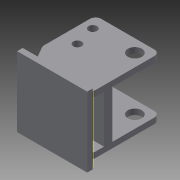
# Autodesk Inventor part: kepala 1 revisi
Saved by Autodesk Inventor 2014 SP2 (Build 180246200, 246)
## iProperties
Created: 2019-06-26
Part Number: kepala 1 revisi
Material: Generic
Document SubType Name: Modeling
Designer: USER PC
Density: 1 g/cm^3
Appearance: Default
Author: USER PC
Autodesk Inventor part; units mm, degrees
ref_plane "YZ Plane" through (0, 0, 0) normal (1, 0, 0) x (0, 1, 0)
ref_plane "XY Plane" through (0, 0, 0) normal (0, 0, 1) x (1, 0, 0)
sketch "Sketch1" plane through (0, 0, 0) normal (0, 0, 1) x (1, 0, 0)
  circle A0 centre (0, 0) radius 15
  circle A1 centre (150, 0) radius 25
  line L0 (-35, 45) -> (-35, -144.3782)
  circle A2 centre (20.0962, -75) radius 15
  line L1 (195, 45) -> (-35, 45)
  line L2 (195, -205) -> (0, -205)
  line L3 (195, -205) -> (195, 45)
  line L4 (0, -205) -> (-35, -144.3782)
  line L5 (0, -205) -> (70, -205) construction
  dimension "d0" = 230
  dimension "d1" = 120
  constraints: 12 end point, 3 centre point, 1 coincident, 1 equal length, 1 horizontal, 1 parallel, 1 perpendicular
  measures "d0" distance of L1.start L0.start
  measures "d1" angle of L5 L4
extrude "Extrusion1" add sketch "Sketch1" along normal blind 210
fillet "Fillet1" radius 20 1 edges at (195, 45, 105)
fillet "Fillet2" radius 20 1 edges at (195, -205, 105)
fillet "Fillet3" radius 20 3 edges at (0, -205, 105) (-35, -144.3782, 105) (-35, 45, 105)
sketch "Sketch3" plane through (195, 25, 210) normal (1, 0, 0) x (0, 0, -1)
  line L0 (0, -210) -> (0, 0) projected
  line L1 (0, 20) -> (0, -230)
  line L2 (0, -230) -> (20, -230)
  line L3 (20, -230) -> (20, -180)
  line L4 (20, -180) -> (190, -180)
  line L5 (190, -180) -> (190, -230)
  line L6 (190, -230) -> (210, -230)
  line L7 (210, -230) -> (210, 20)
  line L8 (210, 20) -> (190, 20)
  line L9 (190, 20) -> (190, -150)
  line L10 (190, -150) -> (20, -150)
  line L11 (20, -150) -> (20, 20)
  line L12 (20, 20) -> (0, 20)
  point P0 (210, -25)
  dimension "d17" = 250
  dimension "d18" = 20
  dimension "d19" = 50
  dimension "d20" = 170
  dimension "d21" = 170
  constraints: 24 end point, 4 perpendicular, 2 parallel, 1 point on line
  measures "d17" distance of L1.start L1.end
  measures "d18" distance of L1.end L2.end
  measures "d19" distance of L2.end L3.end
  measures "d20" distance of L3.end L4.end
  measures "d21" distance of L8.end L9.end
extrude "Extrusion3" cut sketch "Sketch3" against normal blind 230 keep common part
ref_plane "Work Plane1" through (175, -205, 10) normal (0, 1, 0) x (-1, 0, 0)
sketch "Sketch4" plane through (175, -205, 10) normal (0, 1, 0) x (-1, 0, 0)
  line L0 (210, -30) -> (220, -30)
  line L1 (220, -30) -> (220, 220)
  line L2 (220, 220) -> (-30, 220)
  line L3 (-30, 220) -> (-30, -30)
  line L4 (-30, -30) -> (210, -30)
  point P0 (175, -10)
  dimension "d25" = 10
  dimension "d26" = 250
  dimension "d27" = 250
  dimension "d28" = 250
  constraints: 10 end point, 1 parallel
  measures "d25" distance of L0.start L0.end
  measures "d26" distance of L0.end L1.end
  measures "d27" distance of L1.end L2.end
  measures "d28" distance of L2.end L3.end
extrude "Extrusion4" add sketch "Sketch4" against normal blind 20
body "Solid1"
